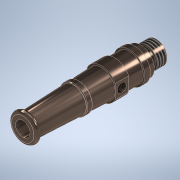
# Autodesk Inventor part: 1. 砲管
Saved by Autodesk Inventor 2022 (Build 260153000, 153)
## iProperties
Created: 2023-05-05
Part Number: 1. 砲管
Material: 一般
Document SubType Name: Modeling
Designer: USER
Density: 1 g/cm^3
Appearance: 砲銅 - 古董色拋光
Author: USER
Autodesk Inventor part; units mm, degrees
ref_plane "YZ Plane" through (0, 0, 0) normal (1, 0, 0) x (0, 1, 0)
ref_plane "XZ Plane" through (0, 0, 0) normal (0, 1, 0) x (-1, 0, 0)
ref_plane "XY Plane" through (0, 0, 0) normal (0, 0, 1) x (1, 0, 0)
sketch "草圖1" plane through (0, 0, 0) normal (1, 0, 0) x (0, 1, 0)
  line L0 (0, 0) -> (0, 6)
  line L1 (0, 6) -> (-14, 6)
  line L2 (-14, 6) -> (-14, -6)
  line L3 (-14, -6) -> (0, -6)
  line L4 (0, -6) -> (0, 0)
  line L5 (0, -6) -> (-12.5, -6)
  line L6 (-12.5, -6) -> (-12.5, -19)
  line L7 (-12.5, -19) -> (0, -19)
  line L8 (0, -19) -> (0, -6)
  line L9 (0, -19) -> (-14, -19)
  line L10 (-14, -19) -> (-14, -24)
  line L11 (-14, -24) -> (0, -24)
  line L12 (0, -24) -> (0, -19)
  line L13 (0, -24) -> (-12.5, -24)
  line L14 (-12.5, -24) -> (-12.5, -29)
  line L15 (-12.5, -29) -> (0, -29)
  line L16 (0, -29) -> (0, -24)
  line L17 (0, -29) -> (-8.5, -29)
  line L18 (-8.5, -29) -> (-8.5, -34)
  line L19 (-8.5, -34) -> (0, -34)
  line L20 (0, -34) -> (0, -29)
  line L21 (0, -34) -> (-10, -34)
  line L22 (-10, -34) -> (-10, -44)
  line L23 (-10, -44) -> (0, -44)
  line L24 (0, -44) -> (0, -34)
  line L25 (0, 6) -> (0, 26)
  line L26 (0, 26) -> (-12.5, 26)
  line L27 (-12.5, 26) -> (-12.5, 31)
  line L28 (-12.5, 31) -> (0, 31)
  line L29 (0, 31) -> (0, 26)
  line L30 (0, 31) -> (0, 71)
  line L31 (0, 71) -> (-12.5, 71)
  line L32 (-12.5, 71) -> (-12.5, 76)
  line L33 (-12.5, 76) -> (0, 76)
  line L34 (0, 76) -> (0, 71)
  line L35 (-12.5, 6) -> (-10, 71)
  point P0 (-11.5385, 31)
  point P1 (-11.7308, 26)
  dimension "d0" = 6
  dimension "d1" = 14
  dimension "d3" = 12
  dimension "d5" = 12.5
  dimension "d6" = 13
  dimension "d7" = 14
  dimension "d8" = 5
  dimension "d9" = 12.5
  dimension "d10" = 5
  dimension "d11" = 8.5
  dimension "d12" = 5
  dimension "d13" = 10
  dimension "d14" = 10
  dimension "d15" = 20
  dimension "d16" = 12.5
  dimension "d17" = 5
  dimension "d18" = 40
  dimension "d19" = 12.5
  dimension "d20" = 5
  dimension "d21" = 10
  dimension "d22" = 12.5
  constraints: 72 end point, 14 parallel, 12 perpendicular, 7 horizontal, 3 point on line, 2 vertical
  measures "d0" distance of L0.start L0.end
  measures "d1" distance of L0.end L1.end
  measures "d3" distance of L1.end L2.end
  measures "d5" distance of L7.end L6.end
  measures "d6" distance of L6.end L5.end
  measures "d7" distance of L11.end L10.end
  measures "d8" distance of L10.end L9.end
  measures "d9" distance of L15.end L14.end
  measures "d10" distance of L14.end L13.end
  measures "d11" distance of L19.end L18.end
  measures "d12" distance of L18.end L17.end
  measures "d13" distance of L23.end L22.end
  measures "d14" distance of L22.end L21.end
  measures "d15" distance of L0.end L25.end
  measures "d16" distance of L27.end L28.end
  measures "d17" distance of L26.end L27.end
  measures "d18" distance of L28.end L30.end
  measures "d19" distance of L32.end L33.end
  measures "d20" distance of L31.end L32.end
  measures "d21" distance of L35.end L30.end
  measures "d22" distance of L35.start L0.end
revolve "迴轉1" add sketch "草圖1" angle 360 about axis through (0, 0, 31) along (0, 0, 1)
chamfer "倒角1" distance 1 angle 45 1 edges at (0, 10, -44)
chamfer "倒角2" distance 0.5 angle 45 2 edges at (0, 12.5, 26) (0, 12.5, 31)
fillet "圓角1" radius 2.5 2 edges at (0, 12.5, 71) (0, 12.5, 76)
sketch "草圖2" plane through (0, 0, 76) normal (0, 0, 1) x (1, 0, 0)
  circle A0 centre (0, 0) radius 11.5385 projected
  circle A1 centre (0, 0) radius 6.5
  dimension "d31" = 13
  constraints: 1 centre point, 1 coincident
  measures "d31" diameter of A1
extrude "擠出1" cut sketch "草圖2" against normal through all contours A1
thread "螺紋1" size "M20x2.5" class "6g" standard "ANSI Metric M Profile" full length
sketch "草圖3" plane through (0, 0, 76) normal (0, 0, 1) x (1, 0, 0)
  line L0 (0, 31.2369) -> (12.5, 31.2369)
  line L1 (12.5, 31.2369) -> (12.5, -26.971)
  line L2 (12.5, -26.971) -> (42.2195, -26.971)
  line L3 (42.2195, -26.971) -> (42.2195, 31.8991)
  line L4 (42.2195, 31.8991) -> (12.5, 31.2369)
  line L5 (0, 31.2369) -> (-12.5, 31.2369)
  line L6 (-12.5, 31.2369) -> (-12.5, -26.3803)
  line L7 (-12.5, -26.3803) -> (-38.1355, -26.3803)
  line L8 (-38.1355, -26.3803) -> (-38.1355, 30.1085)
  line L9 (-38.1355, 30.1085) -> (-12.5, 31.2369)
  point P0 (0, 0)
  dimension "d36" = 12.5
  dimension "d37" = 90
  dimension "d38" = 12.5
  constraints: 20 end point, 5 perpendicular, 2 point on line, 1 horizontal
  measures "d36" distance of L0.start L0.end
  measures "d37" angle of L0 L1
  measures "d38" distance of L0.start L5.end
extrude "擠出2" cut sketch "草圖3" against normal blind 91.75
sketch "草圖4" plane through (12.5, -6.3048, -6) normal (1, 0, 0) x (0, 0, -1)
  circle A0 centre (-6, 6.3048) radius 4
  dimension "d41" = 8
  constraints: 1 centre point, 1 coincident
  measures "d41" diameter of A0
hole "孔1" at (12.5, 0, 0) direction (-1, 0, 0) diameter 8 depth 4 tip angle 118
mirror "鏡射1" about plane through (0, 0, 0) normal (1, 0, 0) of "孔1"
